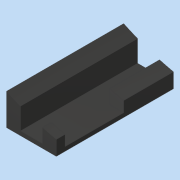
# Autodesk Inventor part: WireGuideToSail2
Saved by Autodesk Inventor 2017 (Build 210142000, 142)
## iProperties
Created: 2018-03-28
Part Number: WireGuideToSail2
Material: ABS Plastic
Document SubType Name: Modeling
Designer: Derek Wider
Density: 1.06 g/cm^3
Appearance: Smooth - Black
Author: Derek Wider
Autodesk Inventor part; units mm, degrees
ref_plane "YZ Plane" through (0, 0, 0) normal (1, 0, 0) x (0, 1, 0)
ref_plane "XZ Plane" through (0, 0, 0) normal (0, 1, 0) x (-1, 0, 0)
sketch "Sketch1" plane through (0, 0, 0) normal (0, 0, 1) x (1, 0, 0)
  line L0 (0, 6.831) -> (0, 0)
  line L1 (0, 0) -> (10.795, 0)
  line L2 (10.795, 0) -> (10.795, 3.175)
  arc A0 (0, 6.831) -> (10.795, 3.175) centre (21.59, 52.8148) ccw
  line L3 (10.795, 3.175) -> (21.59, 3.175) construction
  line L4 (21.59, 3.175) -> (21.59, 2.0148) construction
  arc A1 (10.795, 3.175) -> (21.59, 2.0148) centre (21.59, 52.8148) ccw construction
  dimension "d0" = 50.8
  dimension "d4" = 10.795
  dimension "d12" = 3.175
  dimension "d13" = 10.795
  constraints: 10 end point, 4 point on circle, 3 perpendicular, 2 centre point, 1 coincident, 1 concentric, 1 horizontal, 1 line through centre, 1 point on line, 1 vertical
  measures "d0" radius of A0
  measures "d4" distance of L0.end L1.end
  measures "d12" distance of L1.end L2.end
  measures "d13" distance of L2.end L3.end
extrude "Extrusion1" add sketch "Sketch1" along normal blind 25.4
ref_plane "Work Plane3" through (0, 6.985, 0) normal (0, -1, 0) x (1, 0, 0)
sketch "Sketch4" plane through (0, 6.985, 0) normal (0, -1, 0) x (1, 0, 0)
  line L0 (3.0162, 0) -> (3.0163, 25.4)
  line L1 (0, 25.4) -> (10.795, 25.4) projected
  line L2 (3.0163, 25.4) -> (7.7788, 25.4)
  line L3 (7.7788, 25.4) -> (7.7788, 23.495)
  line L4 (7.7788, 23.495) -> (10.795, 23.495)
  line L5 (10.795, 0) -> (10.795, 25.4) projected
  line L6 (10.795, 23.495) -> (10.795, 10.795)
  line L7 (10.795, 10.795) -> (7.7788, 10.795)
  line L8 (7.7788, 10.795) -> (7.7788, 0)
  line L9 (7.7788, 0) -> (3.0162, 0)
  line L10 (10.795, 0) -> (0, 0) construction
  point P0 (5.3975, 0)
  point P1 (5.3975, 0)
  dimension "d22" = 10.795
  dimension "d23" = 12.7
  dimension "d24" = 4.7625
  constraints: 16 end point, 5 point on line, 4 perpendicular, 2 coincident, 2 midpoint, 1 horizontal, 1 vertical
  measures "d22" distance of L7.end L8.end
  measures "d23" distance of L4.end L6.end
  measures "d24" distance of L0.end L2.end
extrude "Extrusion3" cut sketch "Sketch4" along normal blind 6.096 contours L0 L1 L3 L4 L5 L7 L8 L9
body "Solid1"
